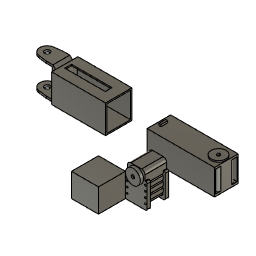
Geometria_motor v1 (Autodesk Fusion 360 design; units mm, degrees)
Autodesk Fusion 360 part; units mm, degrees
note: some values were not read from the file. Set by a fixed rule: which sketch regions a step uses.
sketch "Sketch1" plane through (0, 0, 0) normal (0, 0, 1) x (1, 0, 0)
  line L0 (20, -20) -> (-20, -20)
  line L1 (-20, -20) -> (-20, 20)
  line L2 (-20, 20) -> (20, 20)
  line L3 (20, 20) -> (20, -20)
  line L4 (20, -20) -> (-20, 20) construction
  line L5 (-20, -20) -> (20, 20) construction
  dimension "d1" = 40
  dimension "d2" = 40
  constraint horizontal L0
  constraint perpendicular L0 L1
  constraint parallel L0 L2
  constraint parallel L1 L3
  constraint coincident L4 origin
  constraint coincident L5 origin
  measures "d1" distance of L1.end L2.end
  measures "d2" distance of L0.end L1.end
extrude "Extrude1" add sketch "Sketch1" along normal blind 35 makes body 1
sketch "Sketch2" plane through (0, 0, 0) normal (0, 1, 0) x (1, 0, 0)
  line L0 (39.992, -20) -> (71.992, -20)
  line L1 (71.992, -20) -> (71.992, -70)
  line L2 (71.992, -70) -> (39.992, -70)
  line L3 (39.992, -70) -> (39.992, -20)
  line L4 (55.992, -70) -> (55.992, -58.5)
  line L5 (55.992, -58.5) -> (55.992, -52)
  line L6 (55.992, -52) -> (42.492, -52)
  circle A0 centre (42.492, -52) radius 1.25
  circle A1 centre (69.492, -52) radius 1.25
  circle A2 centre (42.492, -44) radius 1.25
  circle A3 centre (69.492, -44) radius 1.25
  circle A4 centre (42.492, -36) radius 1.25
  circle A5 centre (69.492, -36) radius 1.25
  circle A6 centre (42.492, -28) radius 1.25
  circle A7 centre (69.492, -28) radius 1.25
  dimension "d5" = 32
  dimension "d6" = 50
  dimension "d7" = 11.5
  dimension "d8" = 6.5
  dimension "d9" = 13.5
  dimension "d10" = 2.5
  dimension "d13" = 27
  dimension "d14" = 24
  constraint horizontal L0
  constraint vertical L1
  constraint horizontal L2
  constraint vertical L3
  constraint midpoint L2 L4.start
  constraint perpendicular L2 L4
  constraint vertical L5
  constraint perpendicular L5 L6
  constraint coincident L6.end A0.centre
  measures "d5" distance of L1.end L2.end
  measures "d6" distance of L0.end L1.end
  measures "d7" distance of L4.start L4.end
  measures "d8" distance of L4.end L5.end
  measures "d9" distance of L5.end L6.end
  measures "d10" diameter of A0
extrude "Extrude2" add sketch "Sketch2" along normal blind 5 separate body makes body 2
sketch "Sketch3" plane through (0, 5, 0) normal (0, 1, 0) x (-1, 0, 0)
  circle A0 centre (-42.492, 52) radius 1.25
  circle A1 centre (-42.492, 44) radius 1.25
  circle A2 centre (-69.492, 44) radius 1.25
  circle A3 centre (-69.492, 28) radius 1.25
  circle A4 centre (-42.492, 36) radius 1.25
  circle A5 centre (-69.492, 52) radius 1.25
  circle A6 centre (-42.492, 28) radius 1.25
  circle A7 centre (-69.492, 36) radius 1.25
  line L0 (-39.992, 70) -> (-71.992, 70)
  line L1 (-71.992, 70) -> (-71.992, 20)
  line L2 (-71.992, 20) -> (-39.992, 20)
  line L3 (-39.992, 20) -> (-39.992, 70)
  line L4 (-55.992, 70) -> (-42.992, 70)
  line L5 (-55.992, 70) -> (-55.992, 51)
  line L6 (-42.992, 70) -> (-42.992, 23)
  line L7 (-55.992, 70) -> (-68.992, 70)
  line L8 (-68.992, 70) -> (-68.992, 23)
  line L9 (-68.992, 23) -> (-42.992, 23)
  dimension "d17" = 13
  dimension "d18" = 47
  constraint midpoint L0 L4.start
  constraint coincident L0 L4.end
  constraint parallel L0 L4
  constraint perpendicular L0 L5
  constraint perpendicular L4 L6
  constraint symmetric L4.start L5 L7.start
  constraint symmetric L4.end L5 L7.end
  constraint symmetric L5 L6.end L8.end
  measures "d17" distance of L4.start L4.end
  measures "d18" distance of L4.end L6.end
extrude "Extrude3" add sketch "Sketch3" along normal blind 22 contours A0 A1 A2 A3 A4 A5 A6 A7 L0 L4 L6 L7 L8 L9 bodies 2
sketch "Sketch4" plane through (0, 27, 0) normal (0, 1, 0) x (-1, 0, 0)
  line L0 (-68.992, 26.8544) -> (-68.992, 23)
  line L1 (-68.992, 23) -> (-42.992, 23)
  line L2 (-42.992, 23) -> (-42.992, 26.8544)
  arc A0 (-42.992, 29.1456) -> (-42.992, 26.8544) centre (-42.492, 28) ccw
  line L3 (-42.992, 29.1456) -> (-42.992, 34.8544)
  arc A1 (-42.992, 37.1456) -> (-42.992, 34.8544) centre (-42.492, 36) ccw
  line L4 (-42.992, 37.1456) -> (-42.992, 42.8544)
  arc A2 (-42.992, 45.1456) -> (-42.992, 42.8544) centre (-42.492, 44) ccw
  line L5 (-42.992, 45.1456) -> (-42.992, 50.8544)
  arc A3 (-42.992, 53.1456) -> (-42.992, 50.8544) centre (-42.492, 52) ccw
  line L6 (-42.992, 53.1456) -> (-42.992, 70)
  line L7 (-42.992, 70) -> (-68.992, 70)
  line L8 (-68.992, 70) -> (-68.992, 53.1456)
  arc A4 (-68.992, 50.8544) -> (-68.992, 53.1456) centre (-69.492, 52) ccw
  line L9 (-68.992, 50.8544) -> (-68.992, 45.1456)
  arc A5 (-68.992, 42.8544) -> (-68.992, 45.1456) centre (-69.492, 44) ccw
  line L10 (-68.992, 42.8544) -> (-68.992, 37.1456)
  arc A6 (-68.992, 34.8544) -> (-68.992, 37.1456) centre (-69.492, 36) ccw
  line L11 (-68.992, 34.8544) -> (-68.992, 29.1456)
  arc A7 (-68.992, 26.8544) -> (-68.992, 29.1456) centre (-69.492, 28) ccw
  line L12 (-72.0219, 70) -> (-40, 70)
  line L13 (-40, 70) -> (-40, 20)
  line L14 (-40, 20) -> (-72.0219, 20)
  line L15 (-72.0219, 20) -> (-72.0219, 70)
  constraint horizontal L12
  constraint vertical L13
  constraint horizontal L14
  constraint vertical L15
extrude "Extrude4" add sketch "Sketch4" along normal blind 5 bodies 2
sketch "Sketch5" plane through (0, 0, 0) normal (0, -1, 0) x (1, 0, 0)
  circle A0 centre (42.492, 52) radius 1.25
  circle A1 centre (42.492, 44) radius 1.25
  circle A2 centre (69.492, 44) radius 1.25
  circle A3 centre (69.492, 28) radius 1.25
  circle A4 centre (42.492, 36) radius 1.25
  circle A5 centre (69.492, 52) radius 1.25
  circle A6 centre (42.492, 28) radius 1.25
  circle A7 centre (69.492, 36) radius 1.25
  line L0 (71.992, 70) -> (39.992, 70)
  line L1 (39.992, 70) -> (39.992, 20)
  line L2 (39.992, 20) -> (71.992, 20)
  line L3 (71.992, 20) -> (71.992, 70)
  line L4 (55.992, 70) -> (68.992, 70)
  line L5 (68.992, 70) -> (68.992, 57)
  line L6 (68.992, 70) -> (81, 70)
  line L7 (81, 70) -> (81, 57)
  line L8 (81, 57) -> (68.992, 57)
  line L9 (68.992, 57) -> (68.992, 70)
  line L10 (55.992, 70) -> (55.992, 60)
  line L11 (42.992, 57) -> (42.992, 70)
  line L12 (42.992, 70) -> (30.984, 70)
  line L13 (30.984, 70) -> (30.984, 57)
  line L14 (30.984, 57) -> (42.992, 57)
  dimension "d23" = 13
  dimension "d24" = 13
  constraint midpoint L0 L4.start
  constraint coincident L0 L4.end
  constraint parallel L0 L4
  constraint perpendicular L0 L5
  constraint horizontal L6
  constraint vertical L7
  constraint horizontal L8
  constraint vertical L9
  constraint perpendicular L0 L10
  constraint symmetric L4.end L10 L11.end
  constraint symmetric L6.end L10 L12.end
  constraint symmetric L7.end L10 L13.end
  constraint symmetric L5.end L10 L11.start
  measures "d23" distance of L4.start L4.end
  measures "d24" distance of L4.end L5.end
extrude "Extrude5" cut sketch "Sketch5" against normal blind 33 contours L0 L3 L5 L6 L8 L9 | L3 L6 L7 L8 | L0 L1 L11 L12 L14 | L1 L12 L13 L14 bodies 2
fillet "Fillet1" radius 5 4 edges at (68.992, 16, 70) (42.992, 16, 70) (68.992, 16, 23) (42.992, 16, 23) on bodies 2
fillet "Fillet3" radius 2 8 edges at (72.0219, 29.5, 57) (71.992, 2.5, 57) (40, 29.5, 57) (39.992, 2.5, 57) (40, 29.5, 20) (39.992, 2.5, 20) (71.992, 2.5, 20) (72.0219, 29.5, 20) on bodies 2
sketch "Sketch6" plane through (0, 0, 0) normal (0, -1, 0) x (1, 0, 0)
  circle A0 centre (69.492, 36) radius 1.25
  circle A1 centre (42.492, 28) radius 1.25
  circle A2 centre (69.492, 52) radius 1.25
  circle A3 centre (42.492, 36) radius 1.25
  circle A4 centre (69.492, 28) radius 1.25
  circle A5 centre (69.492, 44) radius 1.25
  circle A6 centre (42.492, 44) radius 1.25
  circle A7 centre (42.492, 52) radius 1.25
  arc A8 (69.992, 20) -> (71.992, 22) centre (69.992, 22) ccw
  line L0 (71.992, 22) -> (71.992, 55)
  arc A9 (71.992, 55) -> (69.992, 57) centre (69.992, 55) ccw
  line L1 (69.992, 57) -> (68.992, 57)
  line L2 (68.992, 57) -> (68.992, 65)
  arc A10 (68.992, 65) -> (63.992, 70) centre (63.992, 65) ccw
  line L3 (63.992, 70) -> (47.992, 70)
  arc A11 (47.992, 70) -> (42.992, 65) centre (47.992, 65) ccw
  line L4 (42.992, 65) -> (42.992, 57)
  line L5 (42.992, 57) -> (41.992, 57)
  arc A12 (41.992, 57) -> (39.992, 55) centre (41.992, 55) ccw
  line L6 (39.992, 55) -> (39.992, 22)
  arc A13 (39.992, 22) -> (41.992, 20) centre (41.992, 22) ccw
  line L7 (41.992, 20) -> (69.992, 20)
  line L8 (55.992, 70) -> (55.992, 58.5)
  circle A14 centre (55.992, 58.5) radius 11
  dimension "d33" = 11.5
  dimension "d34" = 22
  constraint midpoint L3 L8.start
  constraint perpendicular L3 L8
  constraint coincident L8.end A14.centre
  measures "d33" distance of L8.start L8.end
  measures "d34" diameter of A14
extrude "Extrude6" add sketch "Sketch6" along normal blind 5 contours A14 bodies 2
sketch "Sketch7" plane through (0, -5, 0) normal (0, -1, 0) x (1, 0, 0)
  circle A0 centre (55.992, 58.5) radius 11
  circle A1 centre (55.992, 58.5) radius 2.5
  dimension "d37" = 5
  constraint concentric A0 A1
  measures "d37" diameter of A1
extrude "Extrude7" cut sketch "Sketch7" against normal blind 2 contours A1 bodies 2
sketch "Sketch8" plane through (0, 32, 0) normal (0, 1, 0) x (-1, 0, 0)
  arc A0 (-72.0219, 22) -> (-70.0219, 20) centre (-70.0219, 22) ccw
  line L0 (-70.0219, 20) -> (-42, 20)
  arc A1 (-42, 20) -> (-40, 22) centre (-42, 22) ccw
  line L1 (-40, 22) -> (-40, 55)
  arc A2 (-40, 55) -> (-42, 57) centre (-42, 55) ccw
  line L2 (-42, 57) -> (-42.992, 57)
  line L3 (-42.992, 57) -> (-42.992, 65)
  arc A3 (-42.992, 65) -> (-47.992, 70) centre (-47.992, 65) ccw
  line L4 (-47.992, 70) -> (-63.992, 70)
  arc A4 (-63.992, 70) -> (-68.992, 65) centre (-63.992, 65) ccw
  line L5 (-68.992, 65) -> (-68.992, 57)
  line L6 (-68.992, 57) -> (-70.0219, 57)
  arc A5 (-70.0219, 57) -> (-72.0219, 55) centre (-70.0219, 55) ccw
  line L7 (-72.0219, 55) -> (-72.0219, 22)
  line L8 (-55.992, 70) -> (-55.992, 58.5)
  circle A6 centre (-55.992, 58.5) radius 5
  circle A7 centre (-55.992, 58.5) radius 2.5
  dimension "d40" = 11.5
  dimension "d41" = 10
  dimension "d42" = 5
  constraint midpoint L4 L8.start
  constraint perpendicular L4 L8
  constraint coincident L8.end A6.centre
  constraint concentric A6 A7
  measures "d40" distance of L8.start L8.end
  measures "d41" diameter of A6
  measures "d42" diameter of A7
extrude "Extrude8" add sketch "Sketch8" along normal blind 5 contours A6 bodies 2
sketch "Sketch9" plane through (0, 0, 0) normal (0, 1, 0) x (1, 0, 0)
  line L0 (-75, -65) -> (-75, -39)
  line L1 (-75, -65) -> (-87.5, -65)
  line L2 (-87.5, -65) -> (-87.5, -50)
  circle A0 centre (-75, -39) radius 4
  line L3 (-75, -65) -> (-62.5, -65)
  line L4 (-62.5, -65) -> (-62.5, -50)
  line L5 (-62.5, -50) -> (-64.0893, -37.6014)
  line L6 (-87.5, -50) -> (-85.9107, -37.6014)
  arc A1 (-64.0893, -37.6014) -> (-85.9107, -37.6014) centre (-75, -39) ccw
  dimension "d45" = 26
  dimension "d46" = 12.5
  dimension "d47" = 15
  dimension "d48" = 8
  dimension "d49" = 22
  constraint vertical L0
  constraint perpendicular L0 L1
  constraint perpendicular L1 L2
  constraint coincident L0.end A0.centre
  constraint concentric A0 A1
  constraint symmetric L1.start L0 L3.start
  constraint symmetric L0 L1.end L3.end
  constraint symmetric L0 L2.end L4.end
  constraint tangent L5 A1
  constraint tangent L6 A1
  measures "d45" distance of L0.start L0.end
  measures "d46" distance of L0.start L1.end
  measures "d47" distance of L1.end L2.end
  measures "d48" diameter of A0
  measures "d49" diameter of A1
extrude "Extrude9" add sketch "Sketch9" along normal blind 48 separate body makes body 3
sketch "Sketch10" plane through (-87.5, 0, 0) normal (-1, 0, 0) x (0, -1, 0)
  line L0 (0, 50) -> (0, 65)
  line L1 (0, 65) -> (-48, 65)
  line L2 (-48, 65) -> (-48, 50)
  line L3 (-48, 50) -> (0, 50)
  line L4 (-24, 65) -> (-24, 59)
  line L5 (-24, 59) -> (-45, 59)
  line L6 (-45, 59) -> (-45, 25)
  line L7 (-24, 59) -> (-3, 59)
  line L8 (-3, 59) -> (-3, 25)
  line L9 (-45, 25) -> (-3, 25)
  dimension "d52" = 6
  dimension "d53" = 21
  constraint midpoint L1 L4.start
  constraint perpendicular L1 L4
  constraint perpendicular L4 L5
  constraint perpendicular L3 L6
  constraint symmetric L5.start L4 L7.start
  constraint symmetric L4 L5.end L7.end
  constraint symmetric L4 L6.end L8.end
  measures "d52" distance of L4.start L4.end
  measures "d53" distance of L4.end L5.end
extrude "Extrude10" cut sketch "Sketch10" against normal blind 31 contours L3 L6 L8 L9 | L3 L5 L6 L7 L8 bodies 3
chamfer "Chamfer1" distance 5 angle 45 2 edges at (-75, 0, 65) (-75, 48, 65) measured on face at (-70.8333, 32, 65) measured on face at (-74.9004, 48, 57.6629) on bodies 3
shell "Shell1" thickness 2 removed faces 1 at (-79.1667, 31, 59) on bodies 3
sketch "Sketch11" plane through (0, 0, 0) normal (1, 0, 0) x (0, 1, 0)
  line L0 (72.0772, 15.9051) -> (107.0772, 15.9051)
  line L1 (107.0772, 15.9051) -> (107.0772, 53.9051)
  line L2 (107.0772, 53.9051) -> (72.0772, 53.9051)
  line L3 (72.0772, 53.9051) -> (72.0772, 15.9051)
  line L4 (89.5772, 53.9051) -> (89.5772, 15.9051)
  line L5 (73.5772, 50.9051) -> (105.5772, 50.9051)
  line L6 (105.5772, 50.9051) -> (105.5772, 18.9051)
  line L7 (105.5772, 18.9051) -> (73.5772, 18.9051)
  line L8 (73.5772, 18.9051) -> (73.5772, 50.9051)
  line L9 (73.5772, 50.9051) -> (105.5772, 18.9051) construction
  line L10 (105.5772, 50.9051) -> (73.5772, 18.9051) construction
  point P0 (89.5772, 34.9051)
  dimension "d59" = 35
  dimension "d60" = 38
  dimension "d61" = 32
  dimension "d62" = 32
  constraint horizontal L0
  constraint vertical L1
  constraint horizontal L2
  constraint vertical L3
  constraint midpoint L2 L4.start
  constraint midpoint L0 L4.end
  constraint horizontal L5
  constraint perpendicular L5 L6
  constraint parallel L5 L7
  constraint parallel L6 L8
  constraint coincident L9 P0
  constraint coincident L10 P0
  constraint midpoint L4 P0
  measures "d59" distance of L1.end L2.end
  measures "d60" distance of L0.end L1.end
  measures "d61" distance of L5.end L6.end
  measures "d62" distance of L5.start L5.end
extrude "Extrude11" add sketch "Sketch11" along normal blind 100 separate body contours L0 L2 L3 L4 L5 L7 L8 | L0 L1 L2 L4 L5 L6 L7 makes body 4
sketch "Sketch12" plane through (0, 0, 53.9051) normal (0, 0, 1) x (-1, 0, 0)
  line L0 (0, -107.0772) -> (0, -72.0772)
  line L1 (0, -72.0772) -> (-100, -72.0772)
  line L2 (-100, -72.0772) -> (-100, -107.0772)
  line L3 (-100, -107.0772) -> (0, -107.0772)
  line L4 (-100, -89.5772) -> (-88.5, -89.5772)
  circle A0 centre (-88.5, -89.5772) radius 11
  circle A1 centre (-88.5, -89.5772) radius 2.5
  dimension "d65" = 11.5
  dimension "d66" = 22
  dimension "d67" = 5
  constraint midpoint L2 L4.start
  constraint perpendicular L2 L4
  constraint coincident L4.end A0.centre
  constraint concentric A0 A1
  measures "d65" distance of L4.start L4.end
  measures "d66" diameter of A0
  measures "d67" diameter of A1
extrude "Extrude12" add sketch "Sketch12" along normal blind 2 contours A0 bodies 4
sketch "Sketch13" plane through (0, 0, 15.9051) normal (0, 0, -1) x (1, 0, 0)
  line L0 (0, -72.0772) -> (0, -107.0772)
  line L1 (0, -107.0772) -> (100, -107.0772)
  line L2 (100, -107.0772) -> (100, -72.0772)
  line L3 (100, -72.0772) -> (0, -72.0772)
  line L4 (100, -89.5772) -> (88.5, -89.5772)
  circle A0 centre (88.5, -89.5772) radius 5
  circle A1 centre (88.5, -89.5772) radius 2.5
  dimension "d70" = 11.5
  dimension "d71" = 10
  dimension "d72" = 5
  constraint midpoint L2 L4.start
  constraint perpendicular L2 L4
  constraint coincident L4.end A0.centre
  constraint concentric A0 A1
  measures "d70" distance of L4.start L4.end
  measures "d71" diameter of A0
  measures "d72" diameter of A1
extrude "Extrude13" add sketch "Sketch13" along normal blind 2 contours A0 bodies 4
sketch "Sketch14" plane through (100, 0, 0) normal (1, 0, 0) x (0, 1, 0)
  line L0 (105.5772, 18.9051) -> (73.5772, 18.9051)
  line L1 (73.5772, 18.9051) -> (73.5772, 50.9051)
  line L2 (73.5772, 50.9051) -> (105.5772, 50.9051)
  line L3 (105.5772, 50.9051) -> (105.5772, 18.9051)
  line L4 (72.0772, 53.9051) -> (72.0772, 15.9051)
  line L5 (72.0772, 15.9051) -> (107.0772, 15.9051)
  line L6 (107.0772, 15.9051) -> (107.0772, 53.9051)
  line L7 (107.0772, 53.9051) -> (72.0772, 53.9051)
  line L8 (89.5772, 50.9051) -> (76.5772, 50.9051)
  line L9 (76.5772, 50.9051) -> (76.5772, 18.9051)
  line L10 (102.5772, 18.9051) -> (76.5772, 18.9051)
  line L11 (102.5772, 18.9051) -> (102.5772, 50.9051)
  line L12 (89.5772, 50.9051) -> (102.5772, 50.9051)
  dimension "d75" = 13
  dimension "d76" = 26
  constraint midpoint L2 L8.start
  constraint coincident L2 L8.end
  constraint parallel L2 L8
  constraint coincident L0 L9.end
  constraint perpendicular L0 L9
  constraint coincident L0 L10.start
  constraint perpendicular L9 L10
  constraint coincident L2 L11.end
  constraint perpendicular L2 L11
  measures "d75" distance of L8.start L8.end
  measures "d76" distance of L9.end L10.start
extrude "Extrude14" add sketch "Sketch14" against normal blind 50 contours L0 L2 L8 L9 L10 L11 L12 bodies 4
fillet "Fillet4" radius 5 2 edges at (100, 102.5772, 34.9051) (100, 76.5772, 34.9051) on bodies 4
move_body "Move4" bodies 3 to x (0, 0, -1) y (0, 1, 0) z (1, 0, 0) at (-127.5, 0, 2.5)
move_body "Move5" bodies 3 to x (1, 0, 0) y (0, 0, 1) z (0, -1, 0) at (0, 90, 90)
sketch "Sketch19" plane through (-62.5, 0, 0) normal (1, 0, 0) x (0, 1, 0)
  line L0 (25, 133) -> (0, 133)
  line L1 (0, 133) -> (0, 95)
  line L2 (0, 95) -> (25, 95)
  line L3 (25, 95) -> (25, 133)
  line L4 (0, 133) -> (25, 95)
  line L5 (12.5, 114) -> (-7, 114)
  line L6 (-7, 114) -> (-7, 93)
  line L7 (-7, 93) -> (32, 93)
  line L8 (32, 93) -> (32, 135)
  line L9 (32, 135) -> (-7, 135)
  line L10 (-7, 114) -> (-7, 135)
  dimension "d113" = 19.5
  dimension "d114" = 21
  dimension "d115" = 39
  dimension "d116" = 42
  constraint coincident L0.end L1.start
  constraint coincident L2.end L3.start
  constraint midpoint L4 L5.start
  constraint perpendicular L1 L5
  constraint perpendicular L5 L6
  constraint perpendicular L6 L7
  constraint perpendicular L0 L8
  constraint perpendicular L1 L9
  constraint perpendicular L5 L10
  measures "d113" distance of L5.start L5.end
  measures "d114" distance of L5.end L6.end
  measures "d115" distance of L6.end L7.end
  measures "d116" distance of L7.end L8.end
extrude "Extrude19" add sketch "Sketch19" along normal blind 80 contours L0 L3 L4 | L1 L4 L5 | L1 L2 L4 L5 | L6 L7 L8 L9 L10 bodies 3
sketch "Sketch20" plane through (17.5, 0, 0) normal (1, 0, 0) x (0, 1, 0)
  line L0 (-7, 93) -> (32, 93)
  line L1 (32, 93) -> (32, 135)
  line L2 (32, 135) -> (-7, 135)
  line L3 (-7, 135) -> (-7, 93)
  line L4 (12.5, 114) -> (12.5, 133)
  line L5 (12.5, 133) -> (-5, 133)
  line L6 (-5, 133) -> (-5, 95)
  line L7 (-5, 95) -> (30, 95)
  line L8 (30, 95) -> (30, 133)
  line L9 (30, 133) -> (12.5, 133)
  dimension "d120" = 19
  dimension "d121" = 17.5
  dimension "d122" = 38
  dimension "d123" = 35
  constraint perpendicular L2 L4
  constraint perpendicular L3 L5
  constraint perpendicular L5 L6
  constraint perpendicular L6 L7
  constraint perpendicular L7 L8
  measures "d120" distance of L4.start L4.end
  measures "d121" distance of L4.end L5.end
  measures "d122" distance of L5.end L6.end
  measures "d123" distance of L6.end L7.end
extrude "Extrude20" cut sketch "Sketch20" against normal blind 79 contours L5 L6 L7 L8 L9 bodies 3
sketch "Sketch21" plane through (0, 0, 53.9051) normal (0, 0, 1) x (-1, 0, 0)
  line L0 (0, -107.0772) -> (0, -72.0772)
  line L1 (0, -72.0772) -> (-100, -72.0772)
  line L2 (-100, -72.0772) -> (-100, -107.0772)
  line L3 (-100, -107.0772) -> (0, -107.0772)
  circle A0 centre (-88.5, -89.5772) radius 11
  line L4 (0, -89.5772) -> (-5, -89.5772)
  line L5 (-5, -89.5772) -> (-5, -94.5772)
  line L6 (-5, -94.5772) -> (-8, -94.5772)
  line L7 (-5, -84.5772) -> (-8, -84.5772)
  line L8 (-5, -89.5772) -> (-5, -84.5772)
  line L9 (-8, -94.5772) -> (-8, -84.5772)
  dimension "d126" = 5
  dimension "d127" = 5
  dimension "d128" = 3
  constraint midpoint L0 L4.start
  constraint perpendicular L0 L4
  constraint perpendicular L4 L5
  constraint perpendicular L5 L6
  constraint symmetric L5.start L4 L8.start
  constraint symmetric L4 L5.end L7.start
  constraint symmetric L4 L6.end L7.end
  measures "d126" distance of L4.start L4.end
  measures "d127" distance of L4.end L5.end
  measures "d128" distance of L5.end L6.end
extrude "Extrude21" add sketch "Sketch21" along normal blind 3 contours L5 L6 L7 L8 L9 bodies 4
sketch "Sketch22" plane through (0, 0, 135) normal (0, 0, 1) x (-1, 0, 0)
  line L0 (62.5, -32) -> (62.5, 7)
  line L1 (62.5, 7) -> (-17.5, 7)
  line L2 (-17.5, 7) -> (-17.5, -32)
  line L3 (-17.5, -32) -> (62.5, -32)
  line L4 (62.5, -12.5) -> (57.5, -12.5)
  line L5 (57.5, -12.5) -> (57.5, -17.5)
  line L6 (57.5, -17.5) -> (-2.5, -17.5)
  line L7 (57.5, -7.5) -> (-2.5, -7.5)
  line L8 (57.5, -12.5) -> (57.5, -7.5)
  line L9 (-2.5, -17.5) -> (-2.5, -7.5)
  dimension "d131" = 5
  dimension "d132" = 5
  dimension "d133" = 60
  constraint midpoint L0 L4.start
  constraint perpendicular L0 L4
  constraint perpendicular L4 L5
  constraint perpendicular L5 L6
  constraint symmetric L5.start L4 L8.start
  constraint symmetric L4 L5.end L7.start
  constraint symmetric L4 L6.end L7.end
  measures "d131" distance of L4.start L4.end
  measures "d132" distance of L4.end L5.end
  measures "d133" distance of L5.end L6.end
extrude "Extrude22" cut sketch "Sketch22" against normal blind 6 contours L5 L6 L7 L8 L9 bodies 3
equation "d113 = ( 39 / 2 ) * 1 mm"
equation "d114 = ( 42 / 2 ) * 1 mm"
equation "d120 = ( 38 / 2 ) * 1 mm"
equation "d121 = ( 35 / 2 ) * 1 mm"
